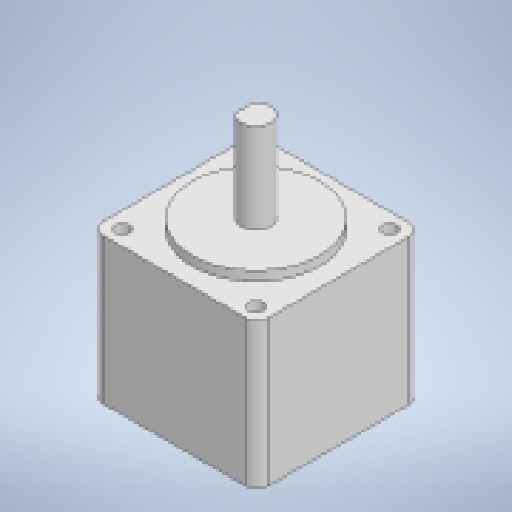
# Autodesk Inventor part: nema 11x25
Saved by Autodesk Inventor 2025 (Build 290162000, 162)
## iProperties
Created: 2025-08-05
Part Number: nema 11x25
Material: 一般
Document SubType Name: Modeling
Designer: gavin
Density: 1 g/cm^3
Appearance: 預設
Author: gavin
Autodesk Inventor part; units mm, degrees
ref_plane "YZ Plane" through (0, 0, 0) normal (1, 0, 0) x (0, 1, 0)
ref_plane "XZ Plane" through (0, 0, 0) normal (0, 1, 0) x (-1, 0, 0)
ref_plane "XY Plane" through (0, 0, 0) normal (0, 0, 1) x (1, 0, 0)
sketch "草圖1" plane through (0, 0, 0) normal (0, 1, 0) x (-1, 0, 0)
  line L0 (-14.25, 14.075) -> (14.25, 14.075)
  line L1 (14.25, 14.075) -> (14.25, -14.075)
  line L2 (14.25, -14.075) -> (-14.25, -14.075)
  line L3 (-14.25, -14.075) -> (-14.25, 14.075)
  line L4 (-14.25, 14.075) -> (14.25, -14.075) construction
  line L5 (14.25, 14.075) -> (-14.25, -14.075) construction
  point P0 (0, 0)
  dimension "d0" = 28.5
  dimension "d1" = 28.15
  constraints: 12 end point, 2 midpoint, 2 parallel, 1 horizontal, 1 perpendicular
  measures "d0" distance of L1.end L2.end
  measures "d1" distance of L0.end L1.end
extrude "擠出1" add sketch "草圖1" along normal blind 25
sketch "草圖2" plane through (0, 25, 0) normal (0, 1, 0) x (1, 0, 0)
  circle A0 centre (0, 0) radius 11
  dimension "d4" = 22
  constraints: 1 centre point, 1 coincident
  measures "d4" diameter of A0
extrude "擠出2" add sketch "草圖2" along normal blind 1.6
sketch "草圖3" plane through (0, 26.6, 0) normal (0, 1, 0) x (1, 0, 0)
  arc A0 (-2, -1.5) -> (-2, 1.5) centre (0, 0) ccw
  line L0 (-2, -1.5) -> (-2, 1.5)
  dimension "d7" = 5
  dimension "d8" = 2
  constraints: 2 end point, 2 point on circle, 1 centre point, 1 coincident, 1 vertical
  measures "d7" diameter of A0
  measures "d8" distance from line of L0 A0.centre
extrude "擠出3" add sketch "草圖3" along normal blind 15.4
sketch "草圖4" plane through (0, 25, 0) normal (0, 1, 0) x (1, 0, 0)
  line L0 (11.5, -11.5) -> (-11.5, -11.5) construction
  line L1 (-11.5, -11.5) -> (-11.5, 11.5) construction
  line L2 (-11.5, 11.5) -> (11.5, 11.5) construction
  line L3 (11.5, 11.5) -> (11.5, -11.5) construction
  arc A0 (-2, -1.5) -> (-2, 1.5) centre (0, 0) ccw construction
  line L4 (11.5, -11.5) -> (-11.5, 11.5) construction
  line L5 (-11.5, -11.5) -> (11.5, 11.5) construction
  circle A1 centre (-11.5, 11.5) radius 1.25
  circle A2 centre (-11.5, -11.5) radius 1.25
  circle A3 centre (11.5, -11.5) radius 1.25
  circle A4 centre (11.5, 11.5) radius 1.25
  dimension "d11" = 23
  dimension "d12" = 23
  dimension "d13" = 2.5
  dimension "d16" = 360
  constraints: 12 end point, 4 centre point, 2 midpoint, 2 parallel, 1 coincident, 1 horizontal, 1 perpendicular, 9 other
  measures "d11" distance of L1.end L2.end
  measures "d12" distance of L0.end L1.end
  measures "d13" diameter of A1
extrude "擠出4" cut sketch "草圖4" against normal blind 3.5
fillet "圓角1" radius 2 4 edges at (14.25, 12.5, 14.075) (14.25, 12.5, -14.075) (-14.25, 12.5, 14.075) (-14.25, 12.5, -14.075)
